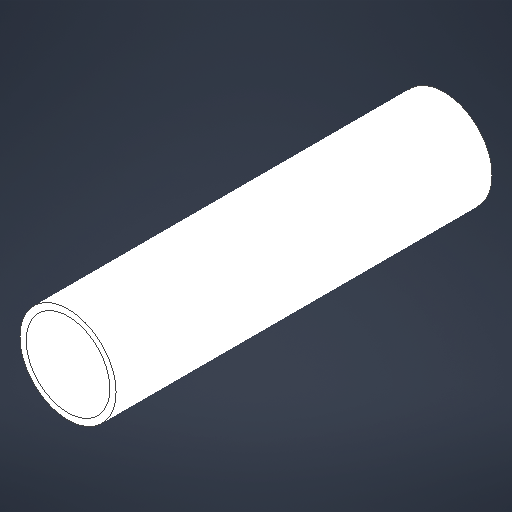
# Autodesk Inventor part: Lifter
Saved by Autodesk Inventor 2026.1 (Build 301233020, 233B)
## iProperties
Created: 2025-11-25
Part Number: Lifter
Material: Generic
Document SubType Name: Modeling
Designer: sarab
Density: 1 g/cm^3
Appearance: Default
Author: sarab
Autodesk Inventor part; units mm, degrees
ref_plane "YZ Plane" through (0, 0, 0) normal (1, 0, 0) x (0, 1, 0)
ref_plane "XZ Plane" through (0, 0, 0) normal (0, 1, 0) x (-1, 0, 0)
ref_plane "XY Plane" through (0, 0, 0) normal (0, 0, 1) x (1, 0, 0)
sketch "Sketch1" plane through (0, 0, 0) normal (0, 0, 1) x (1, 0, 0)
  circle A0 centre (0, 0) radius 10.25
  constraints: 1 centre point, 1 coincident
extrude "Extrusion1" add sketch "Sketch1" along normal blind 80.256
sketch "Sketch2" plane through (0, 0, 80.256) normal (0, 0, 1) x (1, 0, 0)
  circle A0 centre (0, 0) radius 8.9188
  constraints: 1 centre point, 1 coincident
extrude "Extrusion2" cut sketch "Sketch2" against normal blind 78
body "Solid1"
